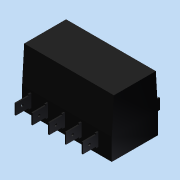
# Autodesk Inventor part: FuseBlock
Saved by Autodesk Inventor 2012 (Build 160160000, 160)
## iProperties
Created: 2012-05-23
Part Number: FuseBlock
Material: Default
Document SubType Name: Modeling
Designer: dgitz
Density: 1 g/cm^3
Author: dgitz
Autodesk Inventor part; units mm, degrees
ref_plane "YZ Plane" through (0, 0, 0) normal (1, 0, 0) x (0, 1, 0)
ref_plane "XZ Plane" through (0, 0, 0) normal (0, 1, 0) x (-1, 0, 0)
sketch "Sketch2" plane through (0, 0, 0) normal (0, 1, 0) x (-1, 0, 0)
  line L0 (-27.178, 13.97) -> (27.178, 13.97)
  line L1 (27.178, 13.97) -> (27.178, -13.97)
  line L2 (27.178, -13.97) -> (-27.178, -13.97)
  line L3 (-27.178, -13.97) -> (-27.178, 13.97)
  line L4 (-27.178, 13.97) -> (27.178, -13.97) construction
  point P0 (0, 0)
  point P1 (0, 0)
  dimension "d0" = 54.356
  dimension "d1" = 27.94
  constraints: 10 end point, 2 parallel, 1 coincident, 1 horizontal, 1 midpoint, 1 perpendicular
  measures "d0" distance between parallel lines of L1 L3
  measures "d1" distance between parallel lines of L2 L0
extrude "Extrusion1" add sketch "Sketch2" along normal blind 12.954
sketch "Sketch3" plane through (-27.178, 0, 13.97) normal (0, 0, 1) x (1, 0, 0)
  line L0 (54.356, 12.954) -> (0, 12.954) projected
  line L1 (0, 0) -> (0, 12.954) projected
  line L2 (54.356, 0) -> (0, 0) projected
  line L3 (4.826, 11.684) -> (5.588, 11.684)
  line L4 (5.588, 11.684) -> (5.588, 3.81)
  line L5 (5.588, 3.81) -> (4.826, 3.81)
  line L6 (4.826, 3.81) -> (4.826, 11.684)
  line L7 (14.986, 11.684) -> (15.748, 11.684)
  line L8 (15.748, 11.684) -> (15.748, 3.81)
  line L9 (15.748, 3.81) -> (14.986, 3.81)
  line L10 (14.986, 3.81) -> (14.986, 11.684)
  line L11 (25.146, 11.684) -> (25.908, 11.684)
  line L12 (25.908, 11.684) -> (25.908, 3.81)
  line L13 (25.908, 3.81) -> (25.146, 3.81)
  line L14 (25.146, 3.81) -> (25.146, 11.684)
  line L15 (35.306, 11.684) -> (36.068, 11.684)
  line L16 (36.068, 11.684) -> (36.068, 3.81)
  line L17 (36.068, 3.81) -> (35.306, 3.81)
  line L18 (35.306, 3.81) -> (35.306, 11.684)
  line L19 (45.466, 11.684) -> (46.228, 11.684)
  line L20 (46.228, 11.684) -> (46.228, 3.81)
  line L21 (46.228, 3.81) -> (45.466, 3.81)
  line L22 (45.466, 3.81) -> (45.466, 11.684)
  point P0 (27.178, 0)
  dimension "d4" = 0.762
  dimension "d5" = 7.874
  dimension "d6" = 1.27
  dimension "d7" = 4.826
  dimension "d10" = 10.16
  constraints: 40 end point, 2 horizontal, 2 parallel, 1 perpendicular, 32 other
  measures "d4" distance between parallel lines of L4 L6
  measures "d5" distance between parallel lines of L3 L5
  measures "d6" distance between parallel lines of L0 L3
  measures "d7" distance between parallel lines of L6 L1
  measures "d10" distance of L3.start L7.start
extrude "Extrusion2" add sketch "Sketch3" along normal blind 9.398
sketch "Sketch4" plane through (-22.352, 3.81, 13.97) normal (-1, 0, 0) x (0, 0, 1)
  line L0 (0, 0) -> (0, 7.874) projected
  line L1 (1.524, 7.874) -> (9.398, 7.874)
  line L2 (9.398, 7.874) -> (9.398, 7.112)
  line L3 (9.398, 7.112) -> (1.524, 7.112)
  line L4 (1.524, 7.112) -> (1.524, 7.874)
  line L5 (9.398, 0) -> (1.524, 0)
  line L6 (1.524, 0) -> (1.524, 0.762)
  line L7 (1.524, 0.762) -> (9.398, 0.762)
  line L8 (9.398, 0.762) -> (9.398, 0)
  circle A0 centre (5.461, 3.937) radius 0.762
  line L9 (9.398, 7.112) -> (1.524, 0.762) construction
  point P0 (-13.97, -3.81)
  dimension "d17" = 6.35
  dimension "d18" = 1.524
  dimension "d19" = 1.524
  constraints: 18 end point, 4 parallel, 2 equal length, 2 horizontal, 2 perpendicular, 1 centre point, 1 coincident, 1 midpoint
  measures "d17" distance between parallel lines of L7 L3
  measures "d18" distance between parallel lines of L4 L0
  measures "d19" diameter of A0
extrude "Extrusion3" cut sketch "Sketch4" against normal up to surface (41.402 mm away)
mirror "Mirror1" about plane through (0, 0, 0) normal (0, 0, 1) of "Extrusion2", "Extrusion3"
sketch "Sketch5" plane through (0, 12.954, 0) normal (0, 1, 0) x (1, 0, 0)
  line L0 (-27.178, -13.97) -> (-27.178, 13.97) projected
  line L1 (27.178, -13.97) -> (-27.178, -13.97) projected
  line L2 (-27.178, 13.97) -> (27.178, 13.97)
  line L3 (27.178, 13.97) -> (27.178, -13.97)
  line L4 (27.178, -13.97) -> (-27.178, -13.97)
  line L5 (-27.178, -13.97) -> (-27.178, 13.97)
  point P0 (0, 0)
  constraints: 8 end point, 2 parallel, 1 horizontal, 1 perpendicular
ref_plane "Work Plane1" through (0, 34.29, 0) normal (0, 1, 0) x (1, 0, 0)
sketch "Sketch6" plane through (0, 34.29, 0) normal (0, 1, 0) x (1, 0, 0)
  line L0 (-27.178, 12.7) -> (27.178, 12.7)
  line L1 (27.178, 12.7) -> (27.178, -12.7)
  line L2 (27.178, -12.7) -> (-27.178, -12.7)
  line L3 (-27.178, -12.7) -> (-27.178, 12.7)
  line L4 (27.178, 12.7) -> (-27.178, -12.7) construction
  point P0 (0, 0)
  point P1 (0, 0)
  point P2 (-27.178, 13.97)
  dimension "d23" = 25.4
  constraints: 10 end point, 2 parallel, 1 coincident, 1 horizontal, 1 midpoint, 1 perpendicular, 1 point on line
  measures "d23" distance between parallel lines of L2 L0
loft "Loft1" add profiles "Sketch5", "Sketch6"
body "Solid1"
